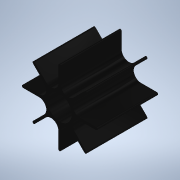
# Autodesk Inventor part: Valvula
Saved by Autodesk Inventor 2020.3 (Build 243373000, 373)
## iProperties
Created: 2021-02-17
Part Number: Valvula
Material: Generic
Document SubType Name: Modeling
Designer: juanp
Density: 1 g/cm^3
Appearance: Glossy - Black
Author: juanp
Autodesk Inventor part; units mm, degrees
ref_plane "YZ Plane" through (0, 0, 0) normal (1, 0, 0) x (0, 1, 0)
ref_plane "XZ Plane" through (0, 0, 0) normal (0, 1, 0) x (-1, 0, 0)
ref_plane "XY Plane" through (0, 0, 0) normal (0, 0, 1) x (1, 0, 0)
sketch "Sketch1" plane through (0, 0, 0) normal (0, 0, 1) x (1, 0, 0)
  circle A0 centre (0, 0) radius 5
  circle A1 centre (0, 0) radius 6
  line L0 (5.9791, 0.5) -> (15, 0.5)
  line L1 (5.9791, -0.5) -> (15, -0.5)
  arc A2 (15, -0.5) -> (15, 0.5) centre (15, 0) ccw
  line L2 (0, 0) -> (15, 0) construction
  line L3 (3.8743, 4.5814) -> (10.253, 10.9602)
  arc A3 (10.9602, 10.253) -> (10.253, 10.9602) centre (10.6066, 10.6066) ccw
  line L4 (4.5814, 3.8743) -> (10.9602, 10.253)
  line L5 (-0.5, 5.9791) -> (-0.5, 15)
  arc A4 (0.5, 15) -> (-0.5, 15) centre (0, 15) ccw
  line L6 (0.5, 5.9791) -> (0.5, 15)
  line L7 (-4.5814, 3.8743) -> (-10.9602, 10.253)
  arc A5 (-10.253, 10.9602) -> (-10.9602, 10.253) centre (-10.6066, 10.6066) ccw
  line L8 (-3.8743, 4.5814) -> (-10.253, 10.9602)
  line L9 (-5.9791, -0.5) -> (-15, -0.5)
  arc A6 (-15, 0.5) -> (-15, -0.5) centre (-15, 0) ccw
  line L10 (-5.9791, 0.5) -> (-15, 0.5)
  circle A7 centre (0, 0) radius 15.5 construction
  line L11 (-3.8743, -4.5814) -> (-10.253, -10.9602)
  arc A8 (-10.9602, -10.253) -> (-10.253, -10.9602) centre (-10.6066, -10.6066) ccw
  line L12 (-4.5814, -3.8743) -> (-10.9602, -10.253)
  line L13 (0.5, -5.9791) -> (0.5, -15)
  arc A9 (-0.5, -15) -> (0.5, -15) centre (0, -15) ccw
  line L14 (-0.5, -5.9791) -> (-0.5, -15)
  line L15 (4.5814, -3.8743) -> (10.9602, -10.253)
  arc A10 (10.253, -10.9602) -> (10.9602, -10.253) centre (10.6066, -10.6066) ccw
  line L16 (3.8743, -4.5814) -> (10.253, -10.9602)
  point P0 (-4.5814, 3.8743)
  point P1 (4.5814, 3.8743)
  point P2 (3.8743, 4.5814)
  point P3 (-3.8743, -4.5814)
  point P4 (-4.5814, -3.8743)
  dimension "d0" = 10
  dimension "d1" = 1
  dimension "d2" = 1
  dimension "d5" = 15
  dimension "d8" = 360
  dimension "d13" = 31
  constraints: 34 end point, 18 point on circle, 11 centre point, 3 coincident, 3 horizontal, 3 tangent, 65 other
  measures "d0" diameter of A0
  measures "d1" radial gap between concentric circles of A1 A0
  measures "d2" distance between parallel lines of L0 L1
  measures "d5" distance of point (0, 0) L2.end
  measures "d13" diameter of A7
extrude "Extrusion1" add sketch "Sketch1" along normal blind 25
fillet "Fillet1" radius 3 16 edges at (5.9791, 0.5, 12.5) (4.5814, 3.8743, 12.5) (-0.5, 5.9791, 12.5) (5.9791, -0.5, 12.5) (-5.9791, 0.5, 12.5) (-5.9791, -0.5, 12.5) (-4.5814, 3.8743, 12.5) (-3.8743, 4.5814, 12.5) (0.5, 5.9791, 12.5) (3.8743, 4.5814, 12.5) (-3.8743, -4.5814, 12.5) (-4.5814, -3.8743, 12.5) (-0.5, -5.9791, 12.5) (0.5, -5.9791, 12.5) (3.8743, -4.5814, 12.5) (4.5814, -3.8743, 12.5)
body "Solid1"
